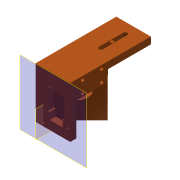
# Autodesk Inventor part: 30_cellSTORM_laserbase_base_v3
Saved by Autodesk Inventor 2019.4 (Build 234330000, 330)
## iProperties
Created: 2021-07-02
Part Number: 30_cellSTORM_laserbase_base_v3
Material: Generic
Document SubType Name: Modeling
Designer: diederichbenedict
Density: 1 g/cm^3
Appearance: Smooth - Light Orange
Mass: 18.3475 g
Surface Area: 86.0517 cm^2
Volume: 18.3475 cm^3
Author: diederichbenedict
Autodesk Inventor part; units mm, degrees
ref_plane "YZ Plane" through (0, 0, 0) normal (1, 0, 0) x (0, 1, 0)
ref_plane "Work Plane1" through (29.8677, -69.0107, 8.183) normal (0, 0, -1) x (-1, 0, 0)
sketch "Sketch1" plane through (29.8677, -69.0107, 8.183) normal (0, 0, -1) x (-1, 0, 0)
  line L0 (2.603, -2) -> (2.603, -17.5) projected
  line L1 (2.603, -17.5) -> (-10.897, -17.5) projected
  line L2 (-10.897, -17.5) -> (-10.897, -2) projected
  line L3 (-10.897, -2) -> (2.603, -2) projected
  circle A0 centre (6.603, -27.5) radius 1 projected
  circle A1 centre (-13.897, -21) radius 1 projected
  circle A2 centre (1.603, 0.5) radius 1 projected
  arc A3 (9.303, -26.8555) -> (8.303, -25.8555) centre (8.303, -26.8555) ccw projected
  line L4 (8.303, -25.8555) -> (5.5653, -25.8555) projected
  arc A4 (4.5653, -24.8555) -> (5.5653, -25.8555) centre (5.5653, -24.8555) ccw projected
  line L5 (4.5653, -24.8555) -> (4.5653, 2) projected
  arc A5 (4.5653, 2) -> (3.5653, 3) centre (3.5653, 2) ccw projected
  line L6 (3.5653, 3) -> (1, 3) projected
  arc A6 (1, 3) -> (0, 2) centre (1, 2) ccw projected
  line L7 (0, 2) -> (0, 1) projected
  arc A7 (-1, 0) -> (0, 1) centre (-1, 1) ccw projected
  line L8 (-1, 0) -> (-12.5347, 0) projected
  line L9 (-12.5347, 0) -> (-12.5347, -18.4723) projected
  arc A8 (-13.5347, -19.4723) -> (-12.5347, -18.4723) centre (-13.5347, -18.4723) ccw projected
  line L10 (-13.5347, -19.4723) -> (-15.397, -19.4723) projected
  arc A9 (-15.397, -19.4723) -> (-16.397, -20.4723) centre (-15.397, -20.4723) ccw projected
  line L11 (-16.397, -20.4723) -> (-16.397, -30) projected
  line L12 (-16.397, -30) -> (9.303, -30) projected
  line L13 (9.303, -30) -> (9.303, -26.8555) projected
  line L14 (-15.7007, 1.7453) -> (12.5653, 1.7453)
  line L15 (12.5653, 1.7453) -> (12.5653, -30.2547)
  line L16 (12.5653, -30.2547) -> (-15.7007, -30.2547)
  line L17 (-15.7007, -30.2547) -> (-15.7007, 1.7453)
  line L18 (1.2141, -1.4589) -> (-9.519, -1.4589)
  line L19 (-9.519, -1.4589) -> (-9.519, -23.1404)
  line L20 (-9.519, -23.1404) -> (1.2141, -23.1404)
  line L21 (1.2141, -23.1404) -> (1.2141, -1.4589)
  ellipse E0 centre (-3.397, -10.2547) end of major axis (-6.4323, -10.2547) minor radius 3.0277 projected
  point P0 (29.8677, 69.0107)
  dimension "d0" = 8
  dimension "d13" = 12
  dimension "d14" = 20
  constraints: 16 end point, 4 parallel, 2 horizontal, 2 perpendicular, 1 other
  measures "d0" distance between parallel lines of L15 L5
  measures "d13" distance from line of L14 point (-3.397, -10.255)
  measures "d14" distance from line of L16 point (-3.397, -10.255)
extrude "Extrusion1" add sketch "Sketch1" along normal blind 5 contours L13 L12 L17 A9 L10 A8 L9 L8 A7 L7 L14 L5 A4 L4 A3 | A3 L4 A4 L5 L14 L15 L16 L17 L12 L13 | L17 L14 L7 A7 L8 L9 A8 L10 A9
sketch "Sketch2" plane through (29.8677, -69.0107, 3.183) normal (0, 0, -1) x (-1, 0, 0)
  line L0 (12.5653, 1.7453) -> (-15.7007, 1.7453) projected
  line L1 (-15.7007, 1.7453) -> (-15.7007, -30.2547) projected
  line L2 (-15.7007, -30.2547) -> (12.5653, -30.2547) projected
  line L3 (12.5653, -30.2547) -> (12.5653, 1.7453) projected
  circle A0 centre (6.603, -27.5) radius 1 projected
  circle A1 centre (-13.897, -21) radius 1 projected
  circle A2 centre (1.603, 0.5) radius 1 projected
  line L4 (1.2141, -17.5) -> (1.2141, -23.1404) projected
  line L5 (1.2141, -23.1404) -> (-9.519, -23.1404) projected
  line L6 (-9.519, -23.1404) -> (-9.519, -17.5) projected
  line L7 (-9.519, -17.5) -> (-10.897, -17.5) projected
  line L8 (-10.897, -17.5) -> (-10.897, -2) projected
  line L9 (-10.897, -2) -> (-9.519, -2) projected
  line L10 (-9.519, -2) -> (-9.519, -1.4589) projected
  line L11 (-9.519, -1.4589) -> (1.2141, -1.4589) projected
  line L12 (1.2141, -1.4589) -> (1.2141, -2) projected
  line L13 (1.2141, -2) -> (2.603, -2) projected
  line L14 (2.603, -2) -> (2.603, -17.5) projected
  line L15 (2.603, -17.5) -> (1.2141, -17.5) projected
  line L16 (-15.7007, 1.7453) -> (12.5653, 1.7453) projected
  line L17 (12.5653, -30.2547) -> (-15.7007, -30.2547) projected
  line L18 (12.5653, 1.7453) -> (6.5653, 1.7453)
  line L19 (6.5653, 1.7453) -> (6.5653, -30.2547)
  line L20 (6.5653, -30.2547) -> (12.5653, -30.2547)
  line L21 (12.5653, -30.2547) -> (12.5653, 1.7453)
  point P0 (29.8677, 69.0107)
  dimension "d6" = 6
  constraints: 8 end point, 2 parallel, 1 horizontal, 1 perpendicular, 1 point on line
  measures "d6" distance of L20.end L19.end
extrude "Extrusion2" add sketch "Sketch2" along normal blind 26 contours L3 L2 L19 A0 L0 | A0 L19 picked at (6.9324, -27.235)
ref_plane "Work Plane5" through (43.2647, -94.0107, -67.7024) normal (0, -1, 0) x (1, 0, 0)
ref_plane "Work Plane6" through (17.2647, -95.0107, -67.7024) normal (0, -1, 0) x (1, 0, 0)
sketch "Sketch7" plane through (17.3024, -67.2655, 8.183) normal (0, 1, 0) x (1, 0, 0)
  line L0 (28.2661, 0) -> (0, 0) projected
  line L1 (28.2661, 0) -> (28.2661, 5) projected
  line L2 (6, 5) -> (28.2661, 5) projected
  line L3 (6, 5) -> (6, 31) projected
  line L4 (0, 31) -> (6, 31) projected
  line L5 (0, 0) -> (0, 31) projected
  line L6 (6, 8.4354) -> (28.2661, 30.7015)
  line L7 (6, 8.4354) -> (37.489, 8.4354) construction
  line L8 (28.2661, 30.7015) -> (6, 30.7015)
  line L9 (6, 30.7015) -> (6, 8.4354)
  point P0 (-17.3024, 8.183)
  dimension "d29" = 45
  dimension "d39" = 0
  constraints: 8 end point, 2 horizontal, 1 equal length, 1 point on line
  measures "d29" angle of L7 L6
  measures "d39" distance from line of L6.end L1
extrude "Extrusion7" add sketch "Sketch7" against normal up to surface (32 mm away) contours L3 L8 L6
sketch "Sketch8" plane through (29.8677, -69.0107, 8.183) normal (0, 0, 1) x (1, 0, 0)
  circle A0 centre (3.397, -10) radius 6 projected
  point P0 (-29.8677, 69.0107)
extrude "Extrusion8" cut sketch "Sketch8" against normal through all
ref_plane "Work Plane7" through (23.3024, -95.0107, 3.183) normal (1, 0, 0) x (0, 0, -1)
sketch "Sketch9" plane through (23.3024, -95.0107, 3.183) normal (1, 0, 0) x (0, 0, -1)
  line L0 (0, 27.7453) -> (3.4354, 27.7453) projected
  line L1 (0, -4.2547) -> (0, -2.4993) projected
  circle A0 centre (13.3978, 16) radius 6 projected
  line L2 (25.7015, 27.7453) -> (25.7015, -4.2547) projected
  line L3 (3.4354, 27.7453) -> (25.7015, 27.7453) projected
  line L4 (3.4354, -4.2547) -> (3.4354, 27.7453) projected
  line L5 (0, 8.5) -> (0, 24) projected
  line L6 (25.7015, 27.7453) -> (0, 27.7453)
  line L7 (0, 27.7453) -> (0, 22.7453)
  line L8 (0, 22.7453) -> (25.7015, 22.7453)
  line L9 (25.7015, 22.7453) -> (25.7015, 27.7453)
  circle A1 centre (5.3442, 25.2453) radius 1.45
  circle A2 centre (20.9266, 25.2453) radius 1.45
  line L10 (0, -0.5007) -> (0, 27.7453) projected
  line L11 (0, -0.5007) -> (0, -2.4993) projected
  line L12 (0, -4.2547) -> (3.4354, -4.2547) projected
  line L13 (3.4354, -4.2547) -> (3.4354, 27.7453) projected
  line L14 (3.4354, -4.2547) -> (25.7015, -4.2547) projected
  line L15 (25.7015, 27.7453) -> (25.7015, -4.2547) projected
  line L16 (25.7015, -4.2547) -> (26, -4.2547) projected
  line L17 (26, 27.7453) -> (26, -4.2547) projected
  line L18 (25.7015, 27.7453) -> (26, 27.7453) projected
  point P0 (3.183, 95.0107)
  dimension "d34" = 5
  dimension "d35" = 2.9
  dimension "d36" = 2.9
  constraints: 8 end point, 2 centre point, 2 parallel, 1 horizontal, 1 perpendicular, 1 point on line
  measures "d34" distance of L7.end L6.end
  measures "d35" diameter of A1
  measures "d36" diameter of A2
extrude "Extrusion9" add sketch "Sketch9" along normal up to surface (22.2661 mm away) contours L0 L4 L8 L5 L7 | L3 L2 L8 L4
sketch "Sketch10" plane through (45.5684, -99.2655, 8.183) normal (1, 0, 0) x (0, 0, -1)
  circle A0 centre (25.9266, 29.5) radius 1.45 projected
  circle A1 centre (10.3442, 29.5) radius 1.45 projected
  line L0 (0, 0) -> (0, 32) projected
  line L1 (0, 0) -> (5, 0) projected
  line L2 (5, 27) -> (5, 0) projected
  line L3 (30.7015, 27) -> (5, 27) projected
  line L4 (30.7015, 32) -> (30.7015, 27) projected
  line L5 (0, 32) -> (30.7015, 32) projected
  line L6 (0, 29.7547) -> (0, 31.7547) projected
  line L7 (0, 31.7547) -> (31, 31.7547)
  line L8 (31, 31.7547) -> (31, 41.7547)
  line L9 (31, 41.7547) -> (0, 41.7547)
  line L10 (0, 41.7547) -> (0, 31.7547)
  line L11 (31, 41.7547) -> (66, 41.7547)
  line L12 (66, 41.7547) -> (66, 36.1607)
  line L13 (66, 36.1607) -> (31, 36.1607)
  line L14 (31, 36.1607) -> (31, 41.7547)
  point P0 (8.183, 99.2655)
  dimension "d40" = 31
  dimension "d41" = 10
  dimension "d42" = 35
  constraints: 16 end point, 4 parallel, 2 horizontal, 2 perpendicular
  measures "d40" distance of L9.end L8.end
  measures "d41" distance of L8.end L7.end
  measures "d42" distance of L12.end L13.end
extrude "Extrusion10" add sketch "Sketch10" against normal up to surface (28.2661 mm away) contours L0 L5 L4 L7 | L10 L9 L8 L7 L4 L5 | L11 L12 L13 L8
sketch "Sketch11" plane through (45.5684, -57.5107, 8.183) normal (0, 1, 0) x (1, 0, 0)
  circle A0 centre (-12.3037, 74.5499) radius 1.4 projected
  circle A1 centre (-12.3037, 46.5499) radius 1.4 projected
  line L0 (-12.3537, 37.4994) -> (-12.3537, 57.4284) construction
  line L1 (-10.6814, 37.4994) -> (-10.6814, 57.4284)
  line L2 (-14.0259, 57.4284) -> (-14.0259, 37.4994)
  arc A2 (-14.0259, 37.4994) -> (-10.6814, 37.4994) centre (-12.3537, 37.4994) ccw
  arc A3 (-10.6814, 57.4284) -> (-14.0259, 57.4284) centre (-12.3537, 57.4284) ccw
  point P0 (-45.5684, 8.183)
  point P1 (-12.3537, 47.4639)
  constraints: 8 end point, 4 point on circle, 4 tangent, 2 centre point, 1 midpoint, 1 parallel, 1 vertical
extrude "Extrusion11" cut sketch "Sketch11" against normal blind 10 contours A2 L2 A3 L1
sketch "Sketch12" plane through (17.3024, -99.2655, -22.817) normal (-1, 0, 0) x (0, 0, 1)
  line L0 (0, 0) -> (0, 36.1607) projected
  line L1 (31, 0) -> (0, 0) projected
  line L2 (31, 41.7547) -> (31, 0) projected
  line L3 (-35, 41.7547) -> (31, 41.7547) projected
  line L4 (-35, 36.1607) -> (-35, 41.7547) projected
  line L5 (0, 36.1607) -> (-35, 36.1607) projected
  circle A0 centre (10.1226, 20.8774) radius 20.8774
  line L6 (24.5, 35.8774) -> (6.5, 35.8774) construction
  line L7 (6.5, 35.8774) -> (6.5, 5.8774) construction
  line L8 (6.5, 5.8774) -> (24.5, 5.8774) construction
  line L9 (24.5, 5.8774) -> (24.5, 35.8774) construction
  line L10 (24.5, 35.8774) -> (6.5, 5.8774) construction
  line L11 (6.5, 35.8774) -> (24.5, 5.8774) construction
  circle A1 centre (27.5, 35.8774) radius 2.45
  circle A2 centre (21.5, 35.8774) radius 2.45
  line L12 (15.5, 25.2048) -> (15.5, 15.1572)
  line L13 (18.2739, 20.8774) -> (11.9104, 20.8774)
  circle A3 centre (3.5, 35.8774) radius 2.45
  circle A4 centre (9.5, 35.8774) radius 2.45
  line L14 (24.5, 5.8774) -> (6.5, 5.8774) construction
  circle A5 centre (27.5, 5.8774) radius 2.45
  circle A6 centre (21.5, 5.8774) radius 2.45
  circle A7 centre (3.5, 5.8774) radius 2.45
  circle A8 centre (9.5, 5.8774) radius 2.45
  point P0 (22.817, 99.2655)
  point P1 (15.5, 20.8774)
  point P2 (0, 5.594)
  dimension "d52" = 18
  dimension "d53" = 30
  dimension "d54" = 4.9
  dimension "d55" = 4.9
  dimension "d59" = 3
  constraints: 18 end point, 9 centre point, 7 symmetric about line, 4 point on line, 3 tangent, 2 horizontal, 2 midpoint, 2 parallel, 1 perpendicular, 1 vertical, 6 other
  measures "d52" distance of L8.end L7.end
  measures "d53" distance of L7.end L6.end
  measures "d54" diameter of A1
  measures "d55" diameter of A2
  measures "d59" distance of L6.start A2.centre
extrude "Extrusion12" cut sketch "Sketch12" against normal blind 3 contours A6 A0 | A0 A6 | A2 A0 | A0 A2 | A1 A0 | A0 A1 | A5 A0 | A0 A5 | A3 | A4 | A7 | A8
sketch "Sketch13" plane through (17.3024, -99.2655, -22.817) normal (-1, 0, 0) x (0, 0, 1)
  circle A0 centre (21.5, 5.8774) radius 2.45 projected
  circle A1 centre (21.5, 35.8774) radius 2.45 projected
  circle A2 centre (3.5, 5.8774) radius 2.45 projected
  circle A3 centre (9.5, 35.8774) radius 2.45 projected
  circle A4 centre (3.5, 35.8774) radius 2.45 projected
  circle A5 centre (9.5, 5.8774) radius 2.45 projected
  circle A6 centre (27.5, 35.8774) radius 2.45 projected
  circle A7 centre (27.5, 5.8774) radius 2.45 projected
  line L0 (0, 0) -> (0, 36.1607) projected
  line L1 (31, 0) -> (0, 0) projected
  line L2 (31, 41.7547) -> (31, 0) projected
  line L3 (-35, 41.7547) -> (31, 41.7547) projected
  line L4 (-35, 36.1607) -> (-35, 41.7547) projected
  line L5 (0, 36.1607) -> (-35, 36.1607) projected
  circle A8 centre (24.3913, 20.8774) radius 3.95
  circle A9 centre (5.641, 20.8774) radius 3.95
  point P0 (22.817, 99.2655)
  dimension "d60" = 7.9
  dimension "d61" = 7.9
  constraints: 2 centre point
  measures "d60" diameter of A8
  measures "d61" diameter of A9
extrude "Extrusion13" cut sketch "Sketch13" against normal blind 4 contours A8 | A9
sketch "Sketch14" plane through (45.5684, -99.2655, 8.183) normal (1, 0, 0) x (0, 0, -1)
  circle A0 centre (25.9266, 29.5) radius 1.65 projected
  circle A1 centre (10.3442, 29.5) radius 1.65 projected
  line L0 (0, 41.7547) -> (0, 0) projected
  line L1 (0, 0) -> (5, 0) projected
  line L2 (5, 27) -> (5, 0) projected
  line L3 (30.7015, 27) -> (5, 27) projected
  line L4 (30.7015, 31.7547) -> (30.7015, 27) projected
  line L5 (30.7015, 31.7547) -> (31, 31.7547) projected
  line L6 (31, 31.7547) -> (31, 36.1607) projected
  line L7 (66, 36.1607) -> (31, 36.1607) projected
  line L8 (66, 41.7547) -> (66, 36.1607) projected
  line L9 (0, 41.7547) -> (66, 41.7547) projected
  circle A2 centre (10.3442, 29.5) radius 1.45 projected
  circle A3 centre (25.9266, 29.5) radius 1.45 projected
  circle A4 centre (25.9266, 38.9577) radius 1.45
  circle A5 centre (10.3442, 38.9577) radius 1.45
  point P0 (8.183, 99.2655)
  dimension "d64" = 2.9
  dimension "d65" = 2.9
  constraints: 2 centre point
  measures "d64" diameter of A4
  measures "d65" diameter of A5
extrude "Extrusion14" cut sketch "Sketch14" against normal blind 20 contours A4 | A5
body "Solid1"
